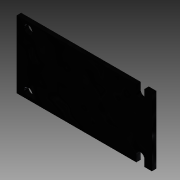
# Autodesk Inventor part: basecam_simpleBCG_32bit_tiny
Saved by Autodesk Inventor 2015 SP1 (Build 190203100, 203)
## iProperties
Created: 2015-08-27
Part Number: basecam_simpleBCG_32bit_tiny
Material: Generic
Document SubType Name: Modeling
Designer: Alexandre Cherpillod
Density: 1 g/cm^3
Appearance: Black
Author: Alexandre Cherpillod
Autodesk Inventor part; units mm, degrees
ref_plane "YZ Plane" through (0, 0, 0) normal (1, 0, 0) x (0, 1, 0)
ref_plane "XZ Plane" through (0, 0, 0) normal (0, 1, 0) x (-1, 0, 0)
ref_plane "XY Plane" through (0, 0, 0) normal (0, 0, 1) x (1, 0, 0)
sketch "Sketch1" plane through (0, 0, 0) normal (0, 1, 0) x (-1, 0, 0)
  line L0 (-50, 0) -> (-50, -25)
  line L1 (0, -25) -> (0, 0)
  circle A0 centre (-4.25, -22.5) radius 1.5
  circle A1 centre (-4.25, -2.5) radius 1.5
  arc A2 (-44.25, -22.5) -> (-47.25, -22.5) centre (-45.75, -22.5) ccw
  arc A3 (-47.25, -2.5) -> (-44.25, -2.5) centre (-45.75, -2.5) ccw
  line L2 (0, -12.5) -> (-50, -12.5) construction
  line L3 (-25, -25) -> (-25, 0) construction
  line L4 (-44.25, -22.5) -> (-44.25, -25)
  line L5 (-47.25, -22.5) -> (-47.25, -25)
  line L6 (-44.25, -2.5) -> (-44.25, 0)
  line L7 (-47.25, -2.5) -> (-47.25, 0)
  line L8 (0, 0) -> (-44.25, 0)
  line L9 (-47.25, 0) -> (-50, 0)
  line L10 (-50, -25) -> (-47.25, -25)
  line L11 (-44.25, -25) -> (0, -25)
  dimension "d0" = 50
  dimension "d1" = 25
  dimension "d2" = 3
  dimension "d3" = 3
  dimension "d4" = 3
  dimension "d5" = 3
  dimension "d7" = 41.5
  dimension "d8" = 20
  dimension "d9" = 10
  dimension "d10" = 20.75
  constraints: 24 end point, 6 perpendicular, 6 point on line, 5 parallel, 4 centre point, 4 point on circle, 2 horizontal, 2 horizontal alignment, 2 midpoint, 2 vertical alignment, 1 tangent
  measures "d0" distance of L1.start L0.end
  measures "d1" distance of L0.end L0.start
  measures "d2" diameter of A0
  measures "d3" diameter of A1
  measures "d4" diameter of A2
  measures "d5" diameter of A3
  measures "d7" distance of A2.centre A0.centre
  measures "d8" distance of A3.centre A2.centre
  measures "d9" distance from line of L2 A0.centre
  measures "d10" distance from line of L3 A2.centre
extrude "Extrusion1" add sketch "Sketch1" against normal blind 1.6
sketch "Sketch2" plane through (0, 0, 0) normal (0, 1, 0) x (1, 0, 0)
  line L0 (38.3, 5.9) -> (28.1, 5.9)
  line L1 (28.1, 5.9) -> (28.1, 10)
  line L2 (28.1, 10) -> (38.3, 10)
  line L3 (38.3, 10) -> (38.3, 5.9)
  line L4 (44.25, 0) -> (0, 0) construction
  line L5 (50, 25) -> (50, 0) construction
  dimension "d13" = 10.2
  dimension "d14" = 4.1
  dimension "d15" = 5.9
  dimension "d16" = 11.7
  constraints: 8 end point, 2 parallel, 1 horizontal, 1 perpendicular
  measures "d13" distance of L0.start L0.end
  measures "d14" distance of L0.end L1.end
  measures "d15" distance between parallel lines of L0 L4
  measures "d16" distance between parallel lines of L5 L3
extrude "Extrusion2" add sketch "Sketch2" along normal blind 2.6
body "Solid1"
